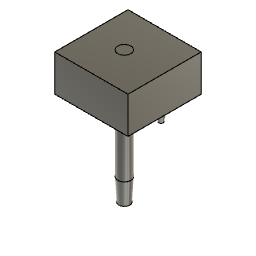
step-1 (Autodesk Fusion 360 design; units mm, degrees)
Autodesk Fusion 360 part; units mm, degrees
box "长方体基本要素1" add length 100 width 100 height 50 placed x (0, -1, 0) y (1, 0, 0) z (0, 0, 1) at (-45, 50, 0) makes body 1
form "造型1" [no effect]
sketch "草图5" plane through (0, 0, 0) normal (0, 1, 0) x (1, 0, 0)
  line L0 (0, 0) -> (0, -150)
  line L1 (0, -150) -> (9, -150)
  line L2 (9, -150) -> (9, 0)
  line L3 (9, 0) -> (7.5, 30)
  line L4 (7.5, 30) -> (0, 30)
  line L5 (0, 30) -> (0, 0)
  constraint coincident L0.start L5.end
  constraint vertical L0
  constraint perpendicular L0 L1
  constraint perpendicular L1 L2
  constraint perpendicular L2 L4
  constraint perpendicular L4 L5
revolve "旋转4" add sketch "草图5" angle 360 about axis through (0, 0, 0) along (0, 0, 1) separate body makes body 2
move_body "移动1" bodies 2 to x (1, 0, 0) y (0, 1, 0) z (0, 0, 1) at (0, 0, -100)
move_body "移动2" bodies 2 to x (1, 0, 0) y (0, 1, 0) z (0, 0, 1) at (-30, 0, 0)
cylinder "圆柱体基本要素3" add diameter 18 height 50 placed x (1, 0, 0) y (0, 1, 0) z (0, 0, 1) at (0, 0, 0) separate body makes body 3
move_body "移动3" bodies 3 to x (1, 0, 0) y (0, 1, 0) z (0, 0, 1) at (0, 0, -10)
sketch "草图8" plane through (0, 0, 0) normal (0, 1, 0) x (1, 0, 0)
  line L0 (53, 7) -> (50, 7)
  line L1 (50, 7) -> (50, -3)
  line L2 (50, -3) -> (55, -3)
  line L3 (55, -3) -> (53, 7)
  constraint horizontal L0
  constraint perpendicular L0 L1
  constraint perpendicular L1 L2
revolve "旋转5" add sketch "草图8" angle 360 about axis through (50, 0, -7) along (0, 0, 1) separate body makes body 4
move_body "移动6" bodies 4 to x (1, 0, 0) y (0, 1, 0) z (0, 0, 1) at (0, 0, -3)
move_body "移动7" bodies 2 to x (1, 0, 0) y (0, 1, 0) z (0, 0, 1) at (30, 0, 0)
move_body "移动8" bodies 3 to x (1, 0, 0) y (0, 1, 0) z (0, 0, 1) at (50, 0, 0)
move_body "移动9" bodies 3 to x (1, 0, 0) y (0, 1, 0) z (0, 0, 1) at (-50, 0, 0)
move_body "移动10" bodies 3 to x (1, 0, 0) y (0, 1, 0) z (0, 0, 1) at (20, 0, 0)
named bodies: "A蓄水箱", "B进水管", "C溢水管", "D出水口"
